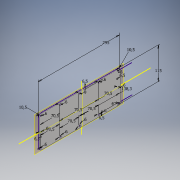
# Autodesk Inventor part: крыша
Saved by Autodesk Inventor 2018.3 (Build 223284000, 284)
## iProperties
Created: 2018-04-26
Part Number: крыша
Material: Типовые
Document SubType Name: Modeling
Designer: kriku
Density: 1 g/cm^3
Appearance: По умолчанию
Mass: 100.473 g
Surface Area: 700.666 cm^2
Volume: 100.473 cm^3
Author: kriku
Autodesk Inventor part; units mm, degrees
sketch "Эскиз1" plane through (0, 0, 0) normal (1, 0, 0) x (0, 1, 0)
  line L0 (-146.2, 57.5) -> (127.8, 57.5)
  line L1 (138.3, 47) -> (138.3, -47)
  line L2 (127.8, -57.5) -> (-146.2, -57.5)
  line L3 (-156.7, -47) -> (-156.7, 47)
  line L4 (-227.1367, 0) -> (250.6977, 0) projected
  arc A0 (-146.2, 57.5) -> (-156.7, 47) centre (-146.2, 47) ccw
  arc A1 (-156.7, -47) -> (-146.2, -57.5) centre (-146.2, -47) ccw
  arc A2 (127.8, -57.5) -> (138.3, -47) centre (127.8, -47) ccw
  arc A3 (138.3, 47) -> (127.8, 57.5) centre (127.8, 47) ccw
  line L5 (-66.5644, 51) -> (182.4356, 51)
  line L6 (131.8, 34) -> (131.8, -35)
  line L7 (182.4356, -51) -> (-66.5644, -51)
  line L8 (-150.2, -35) -> (-150.2, 34)
  circle A4 centre (-79.7, 51) radius 3
  circle A5 centre (-9.2, 51) radius 3
  circle A6 centre (61.3, 51) radius 3
  circle A7 centre (-79.7, -51) radius 3
  circle A8 centre (-9.2, -51) radius 3
  circle A9 centre (61.3, -51) radius 3
  circle A10 centre (131.8, -0.5) radius 3
  circle A11 centre (-150.2, -0.5) radius 3
  line L9 (-150.2, 34) -> (-150.2, 51)
  line L10 (-150.2, 51) -> (-66.5644, 51)
  line L11 (182.4356, 51) -> (131.8, 51)
  line L12 (131.8, 51) -> (131.8, 34)
  line L13 (131.8, -35) -> (131.8, -51)
  line L14 (131.8, -51) -> (181.2224, -51)
  line L15 (-66.5644, -51) -> (-150.2, -51)
  line L16 (-150.2, -36.3739) -> (-150.2, -51)
  circle A12 centre (-150.2, 51) radius 3
  circle A13 centre (-150.2, -51) radius 3
  circle A14 centre (131.8, -51) radius 3
  circle A15 centre (131.8, 51) radius 3
  line L17 (0, -83.5445) -> (0, 83.5445) projected
  point P0 (0, 0)
  dimension "d0" = 115
  dimension "d1" = 295
  dimension "d2" = 10.5
  dimension "d3" = 10.5
  dimension "d7" = 6.5
  dimension "d8" = 6.5
  dimension "d9" = 6.5
  dimension "d10" = 6.5
  dimension "d15" = 6
  dimension "d16" = 6
  dimension "d17" = 6
  dimension "d19" = 6
  dimension "d20" = 6
  dimension "d21" = 6
  dimension "d23" = 6
  dimension "d24" = 6
  dimension "d25" = 70.5
  dimension "d26" = 70.5
  dimension "d27" = 70.5
  dimension "d28" = 6
  dimension "d29" = 6
  dimension "d30" = 6
  dimension "d31" = 6
  dimension "d34" = 70.5
  dimension "d35" = 70.5
  dimension "d36" = 70.5
  dimension "d37" = 138.3
  constraints: 32 end point, 16 centre point, 12 point on line, 8 point on circle, 8 tangent, 5 perpendicular, 4 coincident, 4 parallel, 2 equal radius, 2 horizontal, 2 midpoint, 1 vertical, 1 other
  measures "d0" distance between parallel lines of L2 L0
  measures "d1" distance between parallel lines of L1 L3
  measures "d2" radius of A0
  measures "d3" radius of A3
  measures "d7" distance between parallel lines of L0 L5
  measures "d8" distance between parallel lines of L1 L6
  measures "d9" distance between parallel lines of L2 L7
  measures "d10" distance between parallel lines of L3 L8
  measures "d15" diameter of A4
  measures "d16" diameter of A5
  measures "d17" diameter of A6
  measures "d19" diameter of A7
  measures "d20" diameter of A8
  measures "d21" diameter of A9
  measures "d23" diameter of A10
  measures "d24" diameter of A11
  measures "d25" distance from line of A4.centre L8
  measures "d26" distance of A5.centre A4.centre
  measures "d27" distance of A5.centre A6.centre
  measures "d28" diameter of A12
  measures "d29" diameter of A13
  measures "d30" diameter of A14
  measures "d31" diameter of A15
  measures "d34" distance of A8.centre A7.centre
  measures "d35" distance of A8.centre A9.centre
  measures "d36" distance of L15.end A7.centre
  measures "d37" distance between parallel lines of L1 L17
extrude "Выдавливание1" add sketch "Эскиз1" along normal blind 3.5 contours L0 L17 L5 A5 L10 A4 A12 L9 L8 A11 L4 L3 A0 | L0 A3 L5 A15 A6 L17 | L17 L4 A11 L8 L9 A12 L10 A4 L5 A5 | L5 A6 A15 L12 L6 A10 L4 L17 | L4 A11 L17 L2 A1 L3 | A3 L1 L4 A10 L6 L12 A15 L5 | A5 L5 | L5 A5 | A6 L5 | L5 A6 | L4 A10 L6 L13 A14 L7 A9 L17 | A11 L8 L4 | L4 L8 A11 | A15 L12 L5 | L5 A15 | A11 L8 L4 | L4 L8 A11 | A10 L6 L4 | L4 L6 A10 | L7 A9 A14 A2 L2 L17 | L1 A2 L7 A14 L13 L6 A10 L4 | L12 A15 L5 | L6 A10 L4 | L4 A10 L6 | A9 L7 | L7 A9 | L10 A4 | A4 L10 | A12 L10 L9 | L9 L10 A12 | A14 L7 L13 | L13 L7 A14 | L7 A14 | A8 L7 | L7 A8 | L15 A7 | A7 L15 | A13 L16 L15 | L15 L16 A13
extrude "Выдавливание2" cut sketch "Эскиз1" along normal blind 5 contours A5 L5 | L5 A5 | A6 L5 | L5 A6 | A11 L8 L4 | L4 L8 A11 | A15 L12 L5 | L5 A15 | A11 L8 L4 | L4 L8 A11 | A10 L6 L4 | L4 L6 A10 | L12 A15 L5 | L6 A10 L4 | L4 A10 L6 | A9 L7 | L7 A9 | L10 A4 | A4 L10 | A12 L10 L9 | L9 L10 A12 | A14 L7 L13 | L13 L7 A14 | L7 A14 | A8 L7 | L7 A8 | L15 A7 | A7 L15 | A13 L16 L15 | L15 L16 A13
